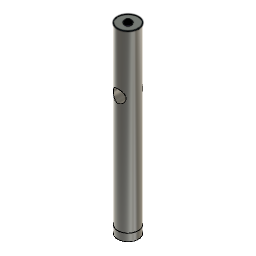
Leg_Link_2 v1 (Autodesk Fusion 360 design; units mm, degrees)
Autodesk Fusion 360 part; units mm, degrees
sketch "Sketch1" plane through (0, 0, 0) normal (0, 0, 1) x (1, 0, 0)
  circle A0 centre (0, 0) radius 4.5
  circle A1 centre (0, 0) radius 1.5
  dimension "d1" = 9
  dimension "d2" = 3
  constraint coincident A0.centre A1.centre
  constraint concentric A0 A1
  measures "d1" diameter of A0
  measures "d2" diameter of A1
extrude "Extrude1" add sketch "Sketch1" against normal blind 76.2 contours A0 | A1 makes body 1
extrude "Extrude2" cut sketch "Sketch1" against normal blind 10 contours A1 bodies 1
sketch "Sketch2" plane through (0, 0, -76.2) normal (0, 0, -1) x (1, 0, 0)
  circle A0 centre (0, 0) radius 4.5
  circle A1 centre (0, 0) radius 1.5
extrude "Extrude3" cut sketch "Sketch2" along normal blind -10 and the other way blind -5 contours A1 bodies 1
ref_plane "WorkPlane1" through (0, 0, 0) normal (0, 1, 0) x (0, 0, 1)
sketch "Sketch3" plane through (0, 0, 0) normal (0, 1, 0) x (1, 0, 0)
  line L0 (4.5, 76.2) -> (-4.5, 76.2)
  line L1 (-4.5, 0) -> (4.5, 0)
  circle A0 centre (0, 25.4) radius 2.75
  line L2 (-4.5, 0) -> (4.5, 0)
  circle A1 centre (0, 81) radius 4.7625
  line L3 (-4.5, 79.4407) -> (-4.5, 76.2)
  arc A2 (-4.5, 79.4407) -> (0, 76.2) centre (0.0531, 81.0184) ccw
  dimension "d10" = 5.5
  dimension "d13" = 25.4
  dimension "d14" = 9.525
  constraint coincident A1 L3.start
  constraint coincident L0.end L3.end
  constraint perpendicular L0 L3
  constraint tangent A1 A2
  constraint midpoint L0 A2.end
  measures "d10" diameter of A0
  measures "d13" distance of A0.centre L2
  measures "d14" diameter of A1
extrude "Extrude4" cut sketch "Sketch3" along normal through all and the other way through all contours A0 bodies 1
revolve "Revolve1" add sketch "Sketch3" angle 360 about axis through (0, 0, 1.75) along (0, 0, 1) separate body contours L0 L3 A2 makes body 2
extrude "Extrude5" cut sketch "Sketch2" along normal blind 5 contours A1 bodies 2
equation "d3 = -25.4 * 3 mm"
equation "d14 = ( ( 3 / 8 ) * 25.4 ) * 1 mm"
